Autodesk Inventor part; units mm, degrees
(part 2 of 2)
  line L377 (-242.6928, 125.0393) -> (-206.7718, 160.9603)
  line L378 (-209.0169, 163.2054) -> (-244.9379, 127.2843)
  arc A322 (-244.9379, 127.2843) -> (-242.6928, 125.0393) centre (-243.8154, 126.1618) ccw
  arc A323 (-206.7718, 160.9603) -> (-209.0169, 163.2054) centre (-207.8943, 162.0828) ccw
  line L379 (-279.7364, 90.2408) -> (-243.8154, 126.1618) construction
  line L380 (-351.5784, 18.3987) -> (-315.6574, 54.3197) construction
  line L381 (-171.9733, 198.0038) -> (-154.0128, 215.9644) construction
  line L382 (-170.8508, 196.8813) -> (-152.8903, 214.8418)
  line L383 (-155.1353, 217.0869) -> (-173.0958, 199.1264)
  arc A324 (-173.0958, 199.1264) -> (-170.8508, 196.8813) centre (-171.9733, 198.0038) ccw
  arc A325 (-152.8903, 214.8418) -> (-155.1353, 217.0869) centre (-154.0128, 215.9644) ccw
  line L384 (-171.9733, 198.0038) -> (-207.8943, 162.0828) construction
  circle A326 centre (-189.9338, 180.0433) radius 25.4 construction
  circle A327 centre (-261.7759, 108.2013) radius 2.159
  circle A328 centre (-189.9338, 180.0433) radius 2.159
  circle A329 centre (-333.6179, 36.3592) radius 2.159
  point P0 (0, 0)
  point P1 (-361.45, 17.8817)
  point P2 (-361.2379, 17.8817)
  point P3 (-359.1386, 16.4954)
  point P4 (-347.4323, 28.2017)
  point P5 (-361.2379, 13.2589)
  point P6 (-339.7697, 24.5506)
  point P7 (-361.3815, 14.2526)
  point P8 (-362.3751, 13.2589)
  point P9 (-273.2207, 32.2327)
  point P10 (-271.4836, 32.2327)
  point P11 (-297.6969, 72.2803)
  point P12 (-225.8548, 144.1223)
  point P13 (-162.993, 206.9841)
  dimension "d0" = 4.318
  dimension "d1" = 25.4
  dimension "d2" = 292.1
  dimension "d3" = 45
  dimension "d10" = 4.318
  dimension "d11" = 15.964
  dimension "d12" = 75.964
  dimension "d13" = 12.7
  dimension "d14" = 12.7
  dimension "d15" = 4.318
  dimension "d16" = 86.424
  dimension "d17" = 26.424
  dimension "d18" = 12.7
  dimension "d19" = 50.8
  dimension "d20" = 203.2
  dimension "d21" = 8
  dimension "d22" = 25.4
  dimension "d23" = 25.4
  dimension "d24" = 4.318
  dimension "d25" = 12.7
  dimension "d26" = 12.7
  dimension "d27" = 41.424
  dimension "d28" = 86.424
  dimension "d29" = 203.2
  dimension "d30" = 12.7
  dimension "d31" = 12.7
  dimension "d32" = 4.318
  dimension "d33" = 18.435
  dimension "d34" = 63.435
  dimension "d35" = 25.4
  dimension "d36" = 19.05
  dimension "d37" = 5.08
  dimension "d38" = 170.18
  dimension "d40" = 25.4
  dimension "d43" = 19.05
  dimension "d44" = 220.98
  dimension "d48" = 50.8
  dimension "d49" = 3.175
  dimension "d50" = 50.8
  dimension "d51" = 3.175
  dimension "d52" = 50.8
  dimension "d53" = 50.8
  dimension "d54" = 3.175
  dimension "d55" = 50.8
  dimension "d56" = 25.4
  dimension "d57" = 4.318
  dimension "d58" = 4.318
  dimension "d59" = 4.318
  constraints: 116 end point, 32 centre point, 25 point on circle, 21 coincident, 18 tangent, 13 parallel, 12 equal radius, 10 midpoint, 8 point on line, 6 perpendicular, 5 horizontal, 4 collinear, 2 equal length, 1 vertical, 1 other
  measures "d0" diameter of A298
  measures "d1" diameter of A299
  measures "d2" distance of L332.start L332.end
  measures "d3" angle of L333 L332
  measures "d10" diameter of A300
  measures "d11" angle of L332 L337
  measures "d12" angle of L337 L341
  measures "d13" distance of L343.end L344.end
  measures "d14" distance of L342.end L343.end
  measures "d15" diameter of A304
  measures "d16" angle of L346 L345
  measures "d17" angle of L332 L346
  measures "d18" distance of L337.end L338.end
  measures "d19" horizontal distance of L332.start L337.end
  measures "d20" distance from line of L350.start L345
  measures "d21" distance between parallel lines of L332 L347
  measures "d22" distance of L347.start L352.end
  measures "d23" distance of L350.start L355.end
  measures "d24" diameter of A308
  measures "d25" distance of L357.end L358.end
  measures "d26" distance of L356.end L357.end
  measures "d27" angle of L332 L360
  measures "d28" angle of L360 L359
  measures "d29" distance from line of L332.start L359
  measures "d30" distance of L362.end L363.end
  measures "d31" distance of L361.end L362.end
  measures "d32" diameter of A312
  measures "d33" angle of L332 L365
  measures "d34" angle of L364 L365
  measures "d35" distance from line of L332.start L364
  measures "d36" diameter of A316
  measures "d37" vertical distance of L332.start L367.start
  measures "d38" radius of A317
  measures "d40" distance of L368.end L332.end
  measures "d43" diameter of A319
  measures "d44" radius of A318
  measures "d48" distance of L373.start L373.end
  measures "d49" diameter of A321
  measures "d50" distance of L376.start L376.end
  measures "d51" diameter of A323
  measures "d52" distance of L373.end L376.start
  measures "d53" distance of L351.start L373.start
  measures "d54" diameter of A325
  measures "d55" diameter of A326
  measures "d56" distance of L383.start L383.end
  measures "d57" diameter of A327
  measures "d58" diameter of A328
  measures "d59" diameter of A329
extrude "Extrusion1" add sketch "Sketch1" along normal blind 3 contours A27 L27 A26 L26 A25 L25 L347 L160 A127 L159 A299 L258 A229 L261 L24 | L24 L347 L25 A25 L26 A26 L27 A27 | A131 L164 A132 L165 A133 L162 A130 L163 | A31 L28 A28 L29 A29 L332 | L332 A29 L30 A30 L31 A31 | L347 L261 A228 L260 A299 L167 A134 L166 A137 L169 L119 L161 A128 L160 L25 A24 L24 | L24 A24 L25 L347 | L347 A299 L260 A228 L261 | L261 A229 L258 A299 L347 | L347 L260 A299 | A299 L258 A226 L259 A227 L260 L347 | L347 A299 L159 A127 L160 | L160 A128 L161 A299 L347 | L260 L347 L111 L332 A231 L263 A230 L262 A233 A299 | A299 L159 L354 L257 A224 L256 A223 L255 L111 L347 L260 A227 L259 A226 L258 | L332 A233 L265 A232 L264 A231 L111 L110 L109 L108 A303 L275 A242 L274 A245 L277 A244 L276 A316 L278 A249 L281 L372 L180 A147 L179 A146 L178 A149 L181 L122 A319 A40 L40 A43 L43 A42 A39 L39 A38 L38 A37 L119 A299 L169 A136 L168 A135 L167 | A299 L354 L159 | L347 L349 L332 L111 | L111 L354 L353 L352 L347 | A299 L169 A137 L166 A134 L167 | L167 A135 L168 A136 L169 A299 | L332 A231 L264 A232 L265 A233 | A233 L262 A230 L263 A231 L332 | L332 L369 L368 A318 L102 A317 L366 L108 A316 A303 L109 L110 L111 | L119 A299 | L354 L255 A223 L256 A224 L257 | L119 A319 L371 A299 | A319 A37 L37 A36 L36 A39 A42 L42 A41 L41 A40 L122 L121 L120 L119 | L119 L120 L121 L122 A319 | A319 A39 L36 A36 L37 A37 | A37 L38 A38 L39 A39 A319 | A319 L122 L372 | A318 L99 A97 L98 A96 L97 L367 A317 L81 A80 L80 A83 L83 L102 | A303 L276 A244 L277 A245 L274 A242 L275 | A318 L97 A96 L98 A97 L99 | A319 A40 L41 A41 L42 A42 | A42 L43 A43 L40 A40 A319 | L181 A149 L178 A146 L179 A147 L180 L372 | A316 L108 | L108 A316 L283 A250 L282 L281 A248 L280 A247 L279 A246 L278 | L83 A83 L80 A80 L81 A317 | L108 L366 L283 A316 | A316 L281 A249 L278 | L278 A246 L279 A247 L280 A248 L281 A316 | A316 L282 A250 L283 | L283 L366 L282 A316 | A316 L282 L366 | L32 A32 L33 A33 L34 A34 L35 A35 | L44 A44 L45 A45 L46 A46 L47 A47 | L84 A84 L85 A85 L86 A86 L87 A87 | L88 A88 L89 A89 L90 A90 L91 A91 | L92 A92 L93 A93 L94 A94 L95 A95 | L170 A138 L171 A139 L172 A140 L173 A141 | L174 A142 L175 A143 L176 A144 L177 A145 | L218 A186 L219 A187 L220 A188 L221 A189 | L222 A190 L223 A191 L224 A192 L225 A193 | L226 A194 L227 A195 L228 A196 L229 A197 | L230 A198 L231 A199 L232 A200 L233 A201 | L266 A234 L267 A235 L268 A236 L269 A237 | L270 A238 L271 A239 L272 A240 L273 A241 | L314 A282 L315 A283 L316 A284 L317 A285 | L318 A286 L319 A287 L320 A288 L321 A289 | L322 A290 L323 A291 L324 A292 L325 A293 | L326 A294 L327 A295 L328 A296 L329 A297
fillet "Fillet2" radius 4.7625 1 edges at (-127.8284, 10.4903, 1.5)
fillet "Fillet3" radius 19.05 6 edges at (-178.6458, 10.4903, 1.5) (-201.9903, 101.726, 1.5) (-361.45, 50.105, 1.5) (-165.8215, 245.7336, 1.5) (-124.2436, 204.1557, 1.5) (-165.1579, 138.5585, 1.5)
body "Solid1"
